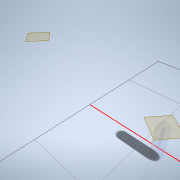
# Autodesk Inventor part: ciecznnieznana
Saved by Autodesk Inventor 2021 (Build 250183000, 183)
## iProperties
Created: 2021-05-23
Part Number: ciecznnieznana
Material: Woda
Document SubType Name: Modeling
Designer: Wojciech Wołczek
Density: 0.9983 g/cm^3
Appearance: Tropikalnie niebieska
Author: Wojciech Wołczek
Autodesk Inventor part; units mm, degrees
ref_plane "YZ Plane" through (0, 0, 0) normal (1, 0, 0) x (0, 1, 0)
ref_plane "XZ Plane" through (0, 0, 0) normal (0, 1, 0) x (-1, 0, 0)
ref_plane "XY Plane" through (0, 0, 0) normal (0, 0, 1) x (1, 0, 0)
ref_plane "Płaszczyzna konstrukcyjna1" through (-75.4734, 102.9977, 14.9612) normal (0, 1, 0) x (0.6304612, 0, -0.7762207)
ref_plane "Płaszczyzna konstrukcyjna2" through (-75.4734, 62.9977, 14.9612) normal (0, 1, 0) x (0.6304612, 0, -0.7762207)
sketch "Szkic1" plane through (-75.4734, 62.9977, 14.9612) normal (0, 1, 0) x (0.6304612, 0, -0.7762207)
  circle A0 centre (0, 0) radius 8
  point P0 (59.1962, -49.1515)
  dimension "d0" = 16
  constraints: 1 centre point
  measures "d0" diameter of A0
extrude "Wyciągnięcie proste1" add sketch "Szkic1" against normal blind 50
fillet "Zaokrąglenie1" radius 7 1 edges at (-80.5171, 12.9977, 21.1709)
sketch "Szkic2" plane through (-75.4734, 62.9977, 14.9612) normal (0, 1, 0) x (1, 0, 0)
  circle A0 centre (0, 0) radius 8 projected
  circle A1 centre (0, 0) radius 1 projected
  circle A2 centre (0, 0) radius 2 projected
  point P0 (75.4734, 14.9612)
extrude "Wyciągnięcie proste2" cut sketch "Szkic2" against normal blind 30 contours A1 | A2
chamfer "Faza1" distance 10 distance2 1 1 edges at (-77.4734, 32.9977, 14.9612) measured on face at (-77.4734, 33.4977, 14.9612)
